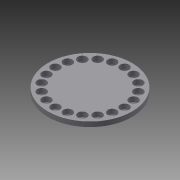
# Autodesk Inventor part: EncoderWheel
Saved by Autodesk Inventor 2014 (Build 180170000, 170)
## iProperties
Created: 2013-05-31
Part Number: EncoderWheel
Material: Generisch
Document SubType Name: Modeling
Designer: hanse
Density: 1 g/cm^3
Appearance: Vorgabe
Author: hanse
Autodesk Inventor part; units mm, degrees
ref_plane "YZ Plane" through (0, 0, 0) normal (1, 0, 0) x (0, 1, 0)
ref_plane "XZ Plane" through (0, 0, 0) normal (0, 1, 0) x (-1, 0, 0)
ref_plane "XY Plane" through (0, 0, 0) normal (0, 0, 1) x (1, 0, 0)
sketch "Skizze1" plane through (0, 0, 0) normal (0, 0, 1) x (1, 0, 0)
  circle A0 centre (0, 0) radius 20
  circle A1 centre (0, 16.4658) radius 2.1227
  circle A2 centre (-5.0882, 15.6599) radius 2.1227
  circle A3 centre (-9.6784, 13.3211) radius 2.1227
  circle A4 centre (-13.3211, 9.6784) radius 2.1227
  circle A5 centre (-15.6599, 5.0882) radius 2.1227
  circle A6 centre (-16.4658, 0) radius 2.1227
  circle A7 centre (-15.6599, -5.0882) radius 2.1227
  circle A8 centre (-13.3211, -9.6784) radius 2.1227
  circle A9 centre (-9.6784, -13.3211) radius 2.1227
  circle A10 centre (-5.0882, -15.6599) radius 2.1227
  circle A11 centre (0, -16.4658) radius 2.1227
  circle A12 centre (5.0882, -15.6599) radius 2.1227
  circle A13 centre (9.6784, -13.3211) radius 2.1227
  circle A14 centre (13.3211, -9.6784) radius 2.1227
  circle A15 centre (15.6599, -5.0882) radius 2.1227
  circle A16 centre (16.4658, 0) radius 2.1227
  circle A17 centre (15.6599, 5.0882) radius 2.1227
  circle A18 centre (13.3211, 9.6784) radius 2.1227
  circle A19 centre (9.6784, 13.3211) radius 2.1227
  circle A20 centre (5.0882, 15.6599) radius 2.1227
  dimension "d0" = 40
  dimension "d3" = 360
  constraints: 21 centre point, 3 coincident, 59 other
  measures "d0" diameter of A0
extrude "Extrusion1" add sketch "Skizze1" along normal blind 2
